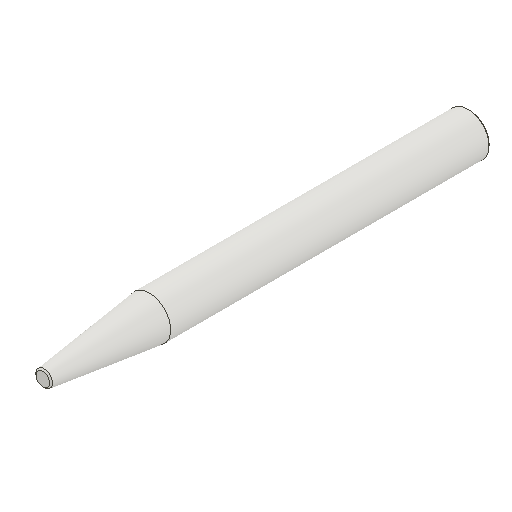
# Autodesk Inventor part: FCT-01-001C
Saved by Autodesk Inventor 2026.1 (Build 301233000, 233)
## iProperties
Company: Delta
Created: 2025-02-17
Part Number: FCT-01-001C
Material: Aço SAE 1045
Document SubType Name: Modeling
Designer: Willian Pinheiro
Density: 7.85 g/cm^3
Appearance: Steel
Project: FCT
Checked By: Antonio Lucas
Description: Eixo Guia 80
Mass: 26.712 g
Surface Area: 20.6578 cm^2
Volume: 3.4028 cm^3
Engr Approved By: Antonio Lucas
Mfg Approved By: Anderson Oliveiro
Dimensões: Ø8 x 80 mm
Total: 2
Author: Willian Pinheiro
Revision Number: 00
Title: FCT
Autodesk Inventor part; units mm, degrees
ref_plane "YZ Plane" through (0, 0, 0) normal (1, 0, 0) x (0, 1, 0)
ref_plane "XZ Plane" through (0, 0, 0) normal (0, 1, 0) x (-1, 0, 0)
ref_plane "XY Plane" through (0, 0, 0) normal (0, 0, 1) x (1, 0, 0)
sketch "Sketch1" plane through (0, 0, 0) normal (0, 0, 1) x (1, 0, 0)
  line L0 (-4.8, 0) -> (0.8, 0) construction
  line L1 (0, -56) -> (0, 56) construction
  line L2 (-4, 40) -> (0, 40)
  line L3 (0, 40) -> (0, -40)
  line L4 (0, -40) -> (-4, -40)
  line L5 (-4, -40) -> (-4, 40)
  line L6 (-1.5443, -40) -> (-4, -20)
  point P0 (0, 0)
  dimension "d0" = 8
  dimension "d1" = 80
  dimension "d13" = 20
  dimension "d14" = 3.0886
  dimension "d17" = 7
  constraints: 10 end point, 3 point on line, 2 parallel, 1 horizontal, 1 perpendicular, 1 other
  measures "d0" diameter of L5 L3
  measures "d1" distance between parallel lines of L4 L2
  measures "d13" vertical distance of L6.start L6.end
  measures "d14" diameter of L6.start L3
  measures "d17" angle of L6 L5
revolve "Revolution1" add sketch "Sketch1" angle 360 about axis through (0, 40, 0) along (0, -1, 0) contours L2 L3 L4 L6 L5
sketch "Sketch2" plane through (0, 40, 0) normal (0, 1, 0) x (1, 0, 0)
  circle A0 centre (0, 0) radius 4
  constraints: 1 centre point, 1 coincident
hole "Hole1" at (0, 40, 0) direction (0, -1, 0) diameter 3.242 depth 15 tip angle 118 thread size "M4x0.7" class "6H" standard "ISO Metric profile"
chamfer "Chamfer1" distance 0.25 angle 45 2 edges at (1.5443, -40, 0) (4, 40, 0)
body "Solid1"
